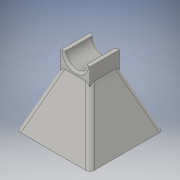
# Autodesk Inventor part: SupportForMouseWire
Saved by Autodesk Inventor 2016 (Build 200138000, 138)
## iProperties
Created: 2015-07-27
Part Number: SupportForMouseWire
Material: Generic
Document SubType Name: Modeling
Designer: steele
Density: 1 g/cm^3
Appearance: Default
Author: steele
Autodesk Inventor part; units mm, degrees
ref_plane "YZ Plane" through (0, 0, 0) normal (1, 0, 0) x (0, 1, 0)
ref_plane "XY Plane" through (0, 0, 0) normal (0, 0, 1) x (1, 0, 0)
sketch "Sketch1" plane through (0, 0, 0) normal (0, 1, 0) x (-1, 0, 0)
  line L0 (-12.7, 12.7) -> (-12.7, -12.7)
  line L1 (-12.7, -12.7) -> (12.7, -12.7)
  line L2 (12.7, -12.7) -> (12.7, 12.7)
  line L3 (12.7, 12.7) -> (-12.7, 12.7)
  line L4 (-12.7, 12.7) -> (12.7, -12.7) construction
  line L5 (-12.7, -12.7) -> (12.7, 12.7) construction
  point P0 (0, 0)
  dimension "base" = 25.4
  constraints: 12 end point, 2 midpoint, 2 parallel, 2 perpendicular, 1 vertical
  measures "base" distance of L2.end L0.start
ref_plane "Work Plane1" through (0, 19.05, 0) normal (0, 1, 0) x (-1, 0, 0)
sketch "Sketch2" plane through (0, 19.05, 0) normal (0, 1, 0) x (-1, 0, 0)
  line L0 (-5.08, 5.08) -> (-5.08, -5.08)
  line L1 (-5.08, -5.08) -> (5.08, -5.08)
  line L2 (5.08, -5.08) -> (5.08, 5.08)
  line L3 (5.08, 5.08) -> (-5.08, 5.08)
  line L4 (-5.08, 5.08) -> (5.08, -5.08) construction
  line L5 (-5.08, -5.08) -> (5.08, 5.08) construction
  point P0 (0, 0)
  dimension "topOfPyramid" = 10.16
  constraints: 12 end point, 2 midpoint, 2 parallel, 2 perpendicular, 1 vertical
  measures "topOfPyramid" distance of L2.end L0.start
loft "Loft1" add profiles "Sketch1", "Sketch2"
sketch "Sketch3" plane through (0, 0, 0) normal (0, 0, 1) x (1, 0, 0)
  arc A0 (-3.81, 24.13) -> (3.81, 24.13) centre (0, 24.13) ccw
  arc A1 (-5.08, 24.13) -> (5.08, 24.13) centre (0, 24.13) ccw
  line L0 (5.08, 19.05) -> (-5.08, 19.05) projected
  line L1 (3.81, 24.13) -> (5.08, 24.13)
  line L2 (-3.81, 24.13) -> (-5.08, 24.13)
  line L3 (-5.08, 24.13) -> (-5.08, 19.05)
  line L4 (5.08, 24.13) -> (5.08, 19.05)
  line L5 (12.7, 0) -> (5.08, 19.05) projected
  line L6 (5.08, 19.05) -> (0, 19.05)
  line L7 (-5.08, 19.05) -> (5.08, 19.05) projected
  line L8 (-5.08, 19.05) -> (0, 19.05)
  point P0 (0, 0)
  dimension "innerDiamForRope" = 7.62
  dimension "centerForRope" = 5.08
  dimension "outsideDiam" = 10.16
  constraints: 12 end point, 4 point on circle, 2 centre point, 1 coincident, 1 collinear, 1 horizontal, 1 midpoint, 1 perpendicular, 1 point on line, 1 tangent
  measures "innerDiamForRope" diameter of A0
  measures "centerForRope" distance from line of L0 A0.centre
  measures "outsideDiam" diameter of A1
extrude "Extrusion1" add sketch "Sketch3" along normal mid plane 10.16
fillet "Fillet3" radius 1.5875 4 edges at (8.89, 9.525, 8.89) (8.89, 9.525, -8.89) (-8.89, 9.525, 8.89) (-8.89, 9.525, -8.89)
fillet "Fillet5" radius 0.7937 2 edges at (0, 20.32, 5.08) (0, 20.32, -5.08)
equation "\"centerForRope\" = 0.5 * outsideDiam"
equation "\"widthOfTop\" = topOfPyramid"
body "Solid1"
